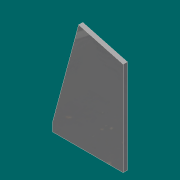
# Autodesk Inventor part: A1-18002-100-54 Tube stop
Saved by Autodesk Inventor 2017 (Build 210142000, 142)
## iProperties
Created: 2018-06-13
Part Number: A1-18002-100-54 Tube stop
Material: Steel, Mild
Document SubType Name: Modeling
Designer: Graeme_Van_Dongen
Density: 7.85 g/cm^3
Appearance: Steel
Author: Graeme_Van_Dongen
Autodesk Inventor part; units mm, degrees
ref_plane "YZ Plane" through (0, 0, 0) normal (1, 0, 0) x (0, 1, 0)
ref_plane "XZ Plane" through (0, 0, 0) normal (0, 1, 0) x (-1, 0, 0)
ref_plane "XY Plane" through (0, 0, 0) normal (0, 0, 1) x (1, 0, 0)
sketch "Sketch1" plane through (0, 0, 0) normal (0, 0, 1) x (1, 0, 0)
  line L0 (0, 0) -> (0, 6.35)
  line L1 (0, 6.35) -> (18.7163, 76.2)
  line L2 (18.7163, 76.2) -> (50.8, 67.6032)
  line L3 (50.8, 67.6032) -> (50.8, 0)
  line L4 (50.8, 0) -> (0, 0)
  dimension "d0" = 50.8
  dimension "d1" = 6.35
  dimension "d2" = 15
  dimension "d3" = 76.2
  constraints: 10 end point, 2 perpendicular, 1 parallel, 1 vertical
  measures "d0" distance of L3.end L0.start
  measures "d1" distance of L0.start L0.end
  measures "d2" angle of L0 L1
  measures "d3" distance from line of L1.end L4
extrude "Extrusion1" add sketch "Sketch1" along normal mid plane 3.048
body "Solid1"
